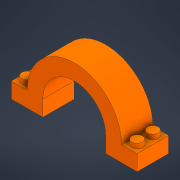
# Autodesk Inventor part: 110033226_ipt_40_背流拱橋
Saved by Autodesk Inventor 2022 (Build 260153000, 153)
## iProperties
Created: 2022-06-26
Part Number: 110033226_ipt_40_背流拱橋
Material: 一般
Document SubType Name: Modeling
Designer: User
Density: 1 g/cm^3
Appearance: 預設
Author: User
Autodesk Inventor part; units mm, degrees
ref_plane "YZ Plane" through (0, 0, 0) normal (1, 0, 0) x (0, 1, 0)
ref_plane "XZ Plane" through (0, 0, 0) normal (0, 1, 0) x (-1, 0, 0)
ref_plane "XY Plane" through (0, 0, 0) normal (0, 0, 1) x (1, 0, 0)
sketch "草圖1" plane through (0, 0, 0) normal (0, 1, 0) x (-1, 0, 0)
  line L0 (0, 0) -> (40, 0)
  line L1 (40, 0) -> (40, -10)
  line L2 (40, -10) -> (0, -10)
  line L3 (0, -10) -> (0, 0)
  line L4 (0, 0) -> (10, 0)
  line L5 (10, 0) -> (10, -10)
  line L6 (10, -10) -> (0, -10)
  line L7 (0, -10) -> (0, 0)
  line L8 (40, 0) -> (30, 0)
  line L9 (30, 0) -> (30, -10)
  line L10 (30, -10) -> (40, -10)
  line L11 (40, -10) -> (40, 0)
  circle A0 centre (7.5, -2.5) radius 1.7
  circle A1 centre (7.5, -7.5) radius 1.7
  circle A2 centre (2.5, -2.5) radius 1.7
  circle A3 centre (2.5, -7.5) radius 1.7
  line L12 (20, 0) -> (20, -10) construction
  circle A4 centre (32.5, -2.5) radius 1.7
  circle A5 centre (32.5, -7.5) radius 1.7
  circle A6 centre (37.5, -2.5) radius 1.7
  circle A7 centre (37.5, -7.5) radius 1.7
  dimension "d0" = 40
  dimension "d1" = 10
  dimension "d2" = 10
  dimension "d3" = 10
  dimension "d4" = 10
  dimension "d5" = 10
  dimension "d6" = 3.4
  dimension "d7" = 2.5
  dimension "d8" = 2.5
  dimension "d11" = 5
  dimension "d14" = 5
  constraints: 26 end point, 8 centre point, 6 parallel, 4 horizontal, 4 symmetric about line, 3 perpendicular, 2 midpoint, 1 vertical, 10 other
  measures "d0" distance of L1.end L2.end
  measures "d1" distance of L0.end L1.end
  measures "d2" distance of L5.end L6.end
  measures "d3" distance of L4.end L5.end
  measures "d4" distance of L10.end L9.end
  measures "d5" distance of L9.end L8.end
  measures "d6" diameter of A0
  measures "d7" distance from line of L5 A0.centre
  measures "d8" distance from line of L0 A0.centre
  measures "d11" distance of A0.centre A1.centre
  measures "d14" distance of A0.centre A2.centre
extrude "擠出1" add sketch "草圖1" along normal blind 5 contours L0 L5 L2 L3 | L0 L1 L2 L9 | A0 | A1 | A2 | A3 | A4 | A5 | A6 | A7
extrude "擠出2" cut sketch "草圖1" along normal blind 1.5 contours A0 | A1 | A2 | A3 | A4 | A5 | A6 | A7
sketch "草圖2" plane through (0, 0, 0) normal (0, 0, 1) x (1, 0, 0)
  line L0 (-40, 0) -> (-30, 0) projected
  line L1 (-30, 0) -> (-30, 5) projected
  line L2 (-40, 5) -> (-30, 5) projected
  line L3 (-40, 0) -> (-40, 5) projected
  line L4 (-10, 0) -> (0, 0) projected
  line L5 (0, 0) -> (0, 5) projected
  line L6 (-10, 5) -> (0, 5) projected
  line L7 (-10, 0) -> (-10, 5) projected
  line L8 (-30, 5) -> (-10, 5) construction
  line L9 (-10, 0) -> (-10, 5) construction
  arc A0 (-10, 5) -> (-30, 5) centre (-20, 5) ccw
  line L10 (-5.8579, 0) -> (-10, 0) construction
  arc A1 (-5, 5) -> (-35, 5) centre (-20, 5) ccw
  dimension "d21" = 5
  constraints: 5 end point, 4 point on circle, 3 midpoint, 2 centre point, 1 horizontal, 1 point on line
  measures "d21" radial gap between concentric circles of A0 A1
extrude "擠出3" add sketch "草圖2" against normal blind 10 contours L2 A1 L6 A0
sketch "草圖3" plane through (0, 5, 0) normal (0, 1, 0) x (1, 0, 0)
  circle A0 centre (-2.5, 7.5) radius 1.7 projected
  point P0 (0, 0)
extrude "擠出4" add sketch "草圖3" along normal blind 1.5
pattern_linear "矩形陣列1" count 2 spacing 5 along (0, 0, 1) count 2 spacing 35 along (-1, 0, 0) of "擠出4"
